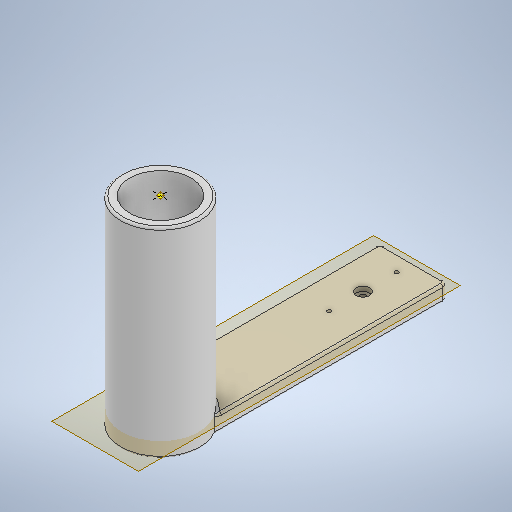
# Autodesk Inventor part: Part5
Saved by Autodesk Inventor 2025.2 (Build 292293000, 293)
## iProperties
Created: 2024-12-14
Part Number: Part5
Material: 一般
Document SubType Name: Modeling
Designer: mahhy
Density: 1 g/cm^3
Appearance: 既定
Mass: 13.5255 g
Surface Area: 84.2705 cm^2
Volume: 13.5255 cm^3
Author: mahhy
## iProperties of the stored document Part5_3D プリント.ipt
Created: 2024-12-19
Part Number: Part5_3D プリント
Material: 一般
Document SubType Name: Modeling
Designer: mahhy
Density: 1 g/cm^3
Appearance: 既定
Author: mahhy
Autodesk Inventor part; units mm, degrees
ref_plane "YZ Plane" through (0, 0, 0) normal (1, 0, 0) x (0, 1, 0)
ref_plane "XZ Plane" through (0, 0, 0) normal (0, 1, 0) x (-1, 0, 0)
ref_plane "XY Plane" through (0, 0, 0) normal (0, 0, 1) x (1, 0, 0)
sketch "スケッチ1" plane through (0, 0, 0) normal (0, 1, 0) x (-1, 0, 0)
  circle A0 centre (0, 0) radius 13.6
  line L0 (14.9651, 22.5) -> (-15.0349, 22.5)
  line L1 (-15.0349, 22.5) -> (-15.0349, -112.5)
  line L2 (-15.0349, -112.5) -> (14.9651, -112.5)
  line L3 (14.9651, -112.5) -> (14.9651, 22.5)
  circle A1 centre (0, -90) radius 1.5
  circle A2 centre (0, 0) radius 17.5
  circle A3 centre (0, -105) radius 0.85
  circle A4 centre (0, -75) radius 0.85
  line L4 (14.9651, 22.5) -> (13.9651, 22.5)
  arc A5 (12.9651, -112.5) -> (14.9651, -110.5) centre (12.9651, -110.5) ccw
  arc A6 (-15.0349, -110.5) -> (-13.0349, -112.5) centre (-13.0349, -110.5) ccw
  arc A7 (14.9651, 20.5) -> (12.9651, 22.5) centre (12.9651, 20.5) ccw
  arc A8 (-13.0349, 22.5) -> (-15.0349, 20.5) centre (-13.0349, 20.5) ccw
  point P0 (-0.0349, 22.5)
  point P1 (0, 13.6)
  point P2 (0, 17.5)
  point P3 (14.9651, -9.0717)
  point P4 (14.9651, 9.0717)
  point P5 (-15.0349, 8.9556)
  point P6 (-15.0349, -8.9556)
  dimension "d0" = 27.2
  dimension "d7" = 35
  dimension "d1" = 30
  dimension "d6" = 3
  dimension "d9" = 5
  dimension "d10" = 90
  dimension "d11" = 135
  dimension "d15" = 15
  dimension "d16" = 15
  dimension "d17" = 1.7
  dimension "d18" = 1.7
  constraints: 10 end point, 9 coincident, 8 point on circle, 8 point on line, 7 centre point, 2 horizontal, 2 parallel, 1 midpoint, 1 perpendicular, 1 vertical alignment, 5 other
  measures "d1" distance of L2.end L1.end
  measures "d6" diameter of A1
  measures "d9" vertical distance of point (-0.035, 22.5) point (0, 17.5)
  measures "d10" distance of A1.centre point (0, 0)
  measures "d11" distance of L2.end L0.start
  measures "d15" distance of point (0, -75) point (0, -90)
  measures "d16" distance of A1.centre point (0, -105)
  measures "d17" diameter of A3
  measures "d18" diameter of A4
extrude "押し出し1" add sketch "スケッチ1" along normal blind 7 contours A2 L3 | L3 A2 L1 | L3 A5 L2 A6 L1 A2 | L1 A2
ref_plane "作業平面1" through (0, 7, 0) normal (0, 1, 0) x (1, 0, 0)
sketch "スケッチ2" plane through (0, 7, 0) normal (0, 1, 0) x (1, 0, 0)
  circle A0 centre (0, 0) radius 17.5
  circle A1 centre (0, 0) radius 13.6
  dimension "d21" = 27.2
  dimension "d22" = 35
  constraints: 3 coincident, 2 centre point
  measures "d21" diameter of A1
  measures "d22" diameter of A0
extrude "押し出し2" add sketch "スケッチ2" along normal blind 82
sketch "スケッチ3" plane through (0, 7, 0) normal (0, 1, 0) x (1, 0, 0)
  circle A0 centre (0, 90) radius 1.5 projected
  circle A1 centre (0, 90) radius 3
  circle A2 centre (0, 90) radius 1.5
  point P0 (0, 0)
  dimension "d31" = 6
  constraints: 2 centre point, 2 coincident, 1 concentric
  measures "d31" diameter of A1
extrude "押し出し3" cut sketch "スケッチ3" against normal blind 2
fillet "フィレット1" radius 1 13 edges at (14.4491, 7, -111.9142) (0.0349, 7, -112.5) (-14.3793, 7, -111.9142) (-14.9651, 7, -59.7858) (15.0349, 7, -59.7278) (14.4491, 0, -111.9142) (0.0349, 0, -112.5) (-14.3793, 0, -111.9142) (-14.9651, 0, -59.7858) (15.0349, 0, -59.7278) (-0.0677, 0, 17.4999) (-17.5, 89, 0) (0.0677, 7, -17.4999)
sketch "スケッチ4" plane through (0, 89, 0) normal (0, 1, 0) x (1, 0, 0)
  point P0 (0, 0)
  point P1 (0, 0)
  constraints: 1 coincident
